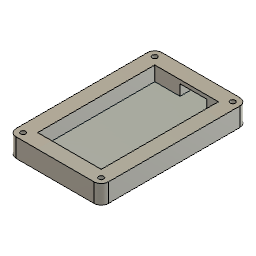
Hackpad v2 (Autodesk Fusion 360 design; units mm, degrees)
Autodesk Fusion 360 part; units mm, degrees
sketch "Sketch1" plane through (0, 0, 0) normal (0, 1, 0) x (1, 0, 0)
  line L0 (22, 40.5) -> (-22, 40.5)
  line L1 (-22, 40.5) -> (-22, -40.5)
  line L2 (-22, -40.5) -> (22, -40.5)
  line L3 (22, -40.5) -> (22, 40.5)
  line L4 (22, 40.5) -> (-22, -40.5) construction
  line L5 (-22, 40.5) -> (22, -40.5) construction
  line L6 (32, 50.5) -> (-32, 50.5)
  line L7 (-32, 50.5) -> (-32, -50.5)
  line L8 (-32, -50.5) -> (32, -50.5)
  line L9 (32, -50.5) -> (32, 50.5)
  line L10 (32, 50.5) -> (-32, -50.5) construction
  line L11 (-32, 50.5) -> (32, -50.5) construction
  line L12 (-32, 50.5) -> (-27, 50.5)
  line L13 (-32, 45.5) -> (-32, 50.5)
  circle A0 centre (-27, 45.5) radius 1.7
  circle A1 centre (-27, 45.5) radius 3
  line L14 (32, 50.5) -> (27, 50.5)
  line L15 (32, 45.5) -> (32, 50.5)
  circle A2 centre (27, 45.5) radius 1.7
  circle A3 centre (27, 45.5) radius 3
  line L16 (32, -50.5) -> (27, -50.5)
  line L17 (32, -45.5) -> (32, -50.5)
  circle A4 centre (27, -45.5) radius 1.7
  circle A5 centre (27, -45.5) radius 3
  line L18 (-32, -50.5) -> (-27, -50.5)
  line L19 (-32, -45.5) -> (-32, -50.5)
  circle A6 centre (-27, -45.5) radius 1.7
  circle A7 centre (-27, -45.5) radius 3
  dimension "d1" = 44
  dimension "d2" = 81
  dimension "d3" = 64
  dimension "d4" = 101
  dimension "d5" = 5
  dimension "d6" = 5
  dimension "d7" = 3.4
  dimension "d8" = 6
  dimension "d9" = 5
  dimension "d10" = 5
  dimension "d11" = 3.4
  dimension "d12" = 6
  dimension "d13" = 5
  dimension "d14" = 5
  dimension "d15" = 3.4
  dimension "d16" = 6
  dimension "d17" = 5
  dimension "d18" = 5
  dimension "d19" = 3.4
  dimension "d20" = 6
  constraint horizontal L0
  constraint perpendicular L0 L1
  constraint parallel L0 L2
  constraint parallel L1 L3
  constraint coincident L4 origin
  constraint coincident L5 origin
  constraint horizontal L6
  constraint perpendicular L6 L7
  constraint parallel L6 L8
  constraint parallel L7 L9
  constraint coincident L10 origin
  constraint coincident L11 origin
  constraint horizontal L12
  constraint vertical L13
  constraint concentric A0 A1
  constraint horizontal L14
  constraint vertical L15
  constraint concentric A2 A3
  constraint horizontal L16
  constraint vertical L17
  constraint concentric A4 A5
  constraint horizontal L18
  constraint vertical L19
  constraint concentric A6 A7
  measures "d1" distance of L1.end L2.end
  measures "d2" distance of L0.end L1.end
  measures "d3" distance of L7.end L8.end
  measures "d4" distance of L6.end L7.end
  measures "d5" distance of L6.end L12.end
  measures "d6" distance of L6.end L13.start
  measures "d7" diameter of A0
  measures "d8" diameter of A1
  measures "d9" distance of L6.start L14.end
  measures "d10" distance of L6.start L15.start
  measures "d11" diameter of A2
  measures "d12" diameter of A3
  measures "d13" distance of L8.end L16.end
  measures "d14" distance of L8.end L17.start
  measures "d15" diameter of A4
  measures "d16" diameter of A5
  measures "d17" distance of L7.end L18.end
  measures "d18" distance of L7.end L19.start
  measures "d19" diameter of A6
  measures "d20" diameter of A7
extrude "Extrude1" add sketch "Sketch1" along normal blind 9.9 from surface at 3.1 contours A1 | A3 | A5 | A7 makes body 1 at (29.9963, 9.7, 45.6495) makes body 2 at (-29.9963, 9.7, 45.6495) makes body 3 at (29.9963, 9.7, -45.3505) makes body 4 at (-29.9963, 9.7, -45.3505)
extrude "Extrude2" add sketch "Sketch1" along normal blind 13 contours L6 L7 L8 L9 L12 L13 L14 L15 L16 L17 L18 L19 bodies 1 2 3 4
extrude "Extrude3" add sketch "Sketch1" along normal blind 3 contours L0 L1 L2 L3 bodies 1
sketch "Sketch2" plane through (0, 3, 0) normal (0, 1, 0) x (-1, 0, 0)
  line L0 (-22, 40.5) -> (-22, -40.5)
  line L1 (-22, -40.5) -> (22, -40.5)
  line L2 (22, -40.5) -> (22, 40.5)
  line L3 (22, 40.5) -> (-22, 40.5)
  line L4 (-22, -40.5) -> (-32, -40.5)
  line L5 (-32, -40.5) -> (-32, -50.5)
  line L6 (-32, -50.5) -> (-22, -50.5)
  line L7 (-22, -50.5) -> (-22, -40.5)
  line L8 (-22, -50.5) -> (-14, -50.5)
  line L9 (-14, -50.5) -> (-14, -40.5)
  line L10 (-14, -40.5) -> (-22, -40.5)
  line L11 (-22, -40.5) -> (-22, -50.5)
  line L12 (-14, -50.5) -> (4.5, -50.5)
  line L13 (4.5, -50.5) -> (4.5, -40.5)
  line L14 (4.5, -40.5) -> (-14, -40.5)
  line L15 (-14, -40.5) -> (-14, -50.5)
  dimension "d28" = 10
  dimension "d29" = 10
  dimension "d30" = 8
  dimension "d31" = 10
  dimension "d32" = 18.5
  dimension "d33" = 10
  constraint horizontal L4
  constraint vertical L5
  constraint horizontal L6
  constraint vertical L7
  constraint coincident L0.end L1.start
  constraint horizontal L8
  constraint vertical L9
  constraint horizontal L10
  constraint vertical L11
  constraint horizontal L12
  constraint vertical L13
  constraint horizontal L14
  constraint vertical L15
  measures "d28" distance of L0.end L4.end
  measures "d29" distance of L0.end L6.end
  measures "d30" distance of L6.end L8.end
  measures "d31" distance of L6.end L0.end
  measures "d32" distance of L8.end L12.end
  measures "d33" distance of L8.end L9.end
extrude "Extrude4" cut sketch "Sketch2" along normal blind 7.5 contours L1 L9 L12 L13 L14 L15 bodies 1
fillet "Fillet1" radius 5 1 edges at (-32, 6.5, -50.5) on bodies 1
fillet "Fillet2" radius 5 1 edges at (32, 6.5, -50.5) on bodies 1
fillet "Fillet3" radius 5 1 edges at (32, 6.5, 50.5) on bodies 1
fillet "Fillet4" radius 5 1 edges at (-32, 6.5, 50.5) on bodies 1
sketch "Sketch3" plane through (0, 3, 0) normal (0, 1, 0) x (-1, 0, 0)
  line L0 (-22, 40.5) -> (-22, -40.5)
  line L1 (-22, -40.5) -> (-14, -40.5)
  line L2 (-14, -40.5) -> (-14, -50.5)
  line L3 (-14, -50.5) -> (4.5, -50.5)
  line L4 (4.5, -50.5) -> (4.5, -40.5)
  line L5 (4.5, -40.5) -> (22, -40.5)
  line L6 (22, -40.5) -> (22, 40.5)
  line L7 (22, 40.5) -> (-22, 40.5)
